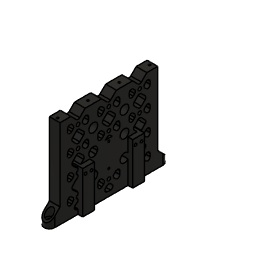
sensors-plate_front-support_rgbd-cameras (Autodesk Fusion 360 design; units mm, degrees)
Autodesk Fusion 360 part; units mm, degrees
note: some values were not read from the file. Set by a fixed rule: which face or edge a step refers to.
(part 1 of 2)
sketch "Sketch1" plane through (0, 90, 0) normal (0, 1, 0) x (-1, 0, 0)
  arc A0 (-180, -120) -> (-165, -135) centre (-165, -120) ccw
  line L0 (-165, -135) -> (165, -135)
  arc A1 (165, -135) -> (180, -120) centre (165, -120) ccw
  line L1 (180, -120) -> (180, 120)
  arc A2 (180, 120) -> (165, 135) centre (165, 120) ccw
  line L2 (165, 135) -> (-165, 135)
  arc A3 (-165, 135) -> (-180, 120) centre (-165, 120) ccw
  line L3 (-180, 120) -> (-180, -120)
  circle A4 centre (165.5, 92) radius 2
  circle A5 centre (-165.5, 92) radius 2 construction
  circle A6 centre (165.5, -92) radius 2
  circle A7 centre (-165.5, -92) radius 2 construction
  line L4 (-178, 131) -> (-180, 131)
  line L5 (-176, -131) -> (-178, -131)
  line L6 (-176, 131) -> (-178, 131)
  line L7 (-178, -131) -> (-180, -131)
  line L8 (-180, 131) -> (-180, -131)
  line L9 (-176, -133) -> (-176, -135)
  line L10 (176, -131) -> (176, -133)
  line L11 (-176, -131) -> (-176, -133)
  line L12 (176, -133) -> (176, -135)
  line L13 (-176, -135) -> (176, -135)
  line L14 (176, 133) -> (176, 135)
  line L15 (-176, 131) -> (-176, 133)
  line L16 (176, 131) -> (176, 133)
  line L17 (-176, 133) -> (-176, 135)
  line L18 (176, 135) -> (-176, 135)
  line L19 (178, -131) -> (180, -131)
  line L20 (176, 131) -> (178, 131)
  line L21 (176, -131) -> (178, -131)
  line L22 (178, 131) -> (180, 131)
  line L23 (180, -131) -> (180, 131)
  circle A8 centre (120, -60) radius 2
  circle A9 centre (0, 120) radius 2
  circle A10 centre (120, 120) radius 2
  circle A11 centre (-120, 0) radius 2
  circle A12 centre (0, -120) radius 2
  circle A13 centre (0, -60) radius 2
  circle A14 centre (165.5, 26.5835) radius 2.5
  circle A15 centre (0, 0) radius 2
  circle A16 centre (60, 120) radius 2
  circle A17 centre (-165.5, -26.5835) radius 2.5 construction
  circle A18 centre (165.5, 78.1855) radius 2.5
  circle A19 centre (120, 0) radius 2
  circle A20 centre (120, -120) radius 2
  circle A21 centre (-60, 60) radius 2
  circle A22 centre (-60, 120) radius 2
  circle A23 centre (-120, -60) radius 2
  circle A24 centre (60, 60) radius 2
  circle A25 centre (0, 60) radius 2
  circle A26 centre (165.5, -26.5835) radius 2.5
  circle A27 centre (60, -60) radius 2
  circle A28 centre (-165.5, 26.5835) radius 2.5 construction
  circle A29 centre (60, 0) radius 2
  circle A30 centre (120, 60) radius 2
  circle A31 centre (165.5, -78.1855) radius 2.5
  circle A32 centre (-120, 60) radius 2
  circle A33 centre (-120, 120) radius 2
  circle A34 centre (-60, -120) radius 2
  circle A35 centre (-165.5, 78.1855) radius 2.5 construction
  circle A36 centre (-120, -120) radius 2
  circle A37 centre (-60, 0) radius 2
  circle A38 centre (60, -120) radius 2
  circle A39 centre (-165.5, -78.1855) radius 2.5 construction
  circle A40 centre (-60, -60) radius 2
  line L24 (176, -131) -> (176, 131)
  line L25 (176, -131) -> (-176, -131)
  line L26 (-176, -131) -> (-176, 131)
  line L27 (-176, 131) -> (176, 131)
  circle A41 centre (-165.5, -92) radius 9
  circle A42 centre (-165.5, 92) radius 9
  circle A43 centre (-165.5, -92) radius 2.25
  circle A44 centre (-165.5, 92) radius 2.25
  line L28 (-156.5, -92) -> (-156.5, 92)
  line L29 (-174.5, 92) -> (-174.5, -92)
  circle A45 centre (-165.5, -78.1855) radius 1.75
  circle A46 centre (-165.5, -26.5835) radius 1.75
  circle A47 centre (-165.5, 26.5835) radius 1.75
  circle A48 centre (-165.5, 78.1855) radius 1.75
  dimension "d15" = 18
  dimension "d17" = 4.5
  dimension "d19" = 3.5
  constraint coincident L10.start L21.start
  constraint coincident L16.start L20.start
  constraint coincident L5.start L11.start
  constraint coincident L6.start L15.start
  constraint concentric A7 A41
  constraint concentric A5 A42
  constraint concentric A41 A43
  constraint concentric A42 A44
  constraint coincident A41 L28.start
  constraint coincident A42 L28.end
  constraint tangent A41 L28
  constraint tangent A42 L28
  constraint coincident A42 L29.start
  constraint coincident A41 L29.end
  constraint tangent A42 L29
  constraint tangent A41 L29
  constraint concentric A39 A45
  constraint concentric A17 A46
  constraint concentric A28 A47
  constraint concentric A35 A48
  constraint equal A45 A46
  constraint equal A45 A47
  constraint equal A45 A48
  constraint equal A41 A42
  constraint equal A43 A44
  measures "d15" diameter of A41
  measures "d17" diameter of A43
  measures "d19" diameter of A45
extrude "Extrude1" add sketch "Sketch1" along normal blind 8 contours A41 | A41 A42 L28 L29 | A42
sketch "Sketch2" plane through (0, 98, 0) normal (0, 1, 0) x (-1, 0, 0)
  circle A0 centre (-165.5, -78.1855) radius 1.75
  circle A1 centre (-165.5, -26.5835) radius 1.75
  circle A2 centre (-165.5, 92) radius 2.25
  circle A3 centre (-165.5, 78.1855) radius 1.75
  circle A4 centre (-165.5, -92) radius 2.25
  circle A5 centre (-165.5, 26.5835) radius 1.75
  line L0 (-174.5, 92) -> (-174.5, -92)
  arc A6 (-174.5, -92) -> (-156.5, -92) centre (-165.5, -92) ccw
  line L1 (-156.5, -92) -> (-156.5, 92)
  arc A7 (-156.5, 92) -> (-174.5, 92) centre (-165.5, 92) ccw
  circle A8 centre (-165.5, -92) radius 9 construction
  line L2 (-165.5, -92) -> (-165.5, -83) construction
  line L3 (-165.5, -83) -> (-156.5, -83)
  line L4 (-165.5, -83) -> (-174.5, -83)
  line L5 (-156.5, 0) -> (-174.5, 0) construction
  line L6 (-156.5, 83) -> (-174.5, 83)
  constraint concentric A4 A8
  constraint coincident A6.end A8
  constraint coincident A4.centre A6.centre
  constraint coincident A8 L2.end
  constraint vertical L2
  constraint coincident L1 L3.end
  constraint perpendicular L1 L3
  constraint coincident L0 L4.end
  constraint perpendicular L0 L4
  constraint midpoint L1 L5.start
  constraint midpoint L0 L5.end
  constraint coincident L1 L6.start
  constraint coincident L0 L6.end
  constraint perpendicular L0 L6
extrude "Extrude2" add sketch "Sketch2" along normal blind 142 contours L0 L1 L3 L4 L6
sketch "Sketch3" plane through (0, 90, 0) normal (0, -1, 0) x (1, 0, 0)
  circle A0 centre (165.5, -78.1855) radius 1.75
  circle A1 centre (165.5, -26.5835) radius 1.75
  circle A2 centre (165.5, 92) radius 2.25
  circle A3 centre (165.5, 78.1855) radius 1.75
  circle A4 centre (165.5, -92) radius 2.25
  circle A5 centre (165.5, 26.5835) radius 1.75
  line L0 (174.5, -92) -> (174.5, 92)
  arc A6 (174.5, 92) -> (156.5, 92) centre (165.5, 92) ccw
  line L1 (156.5, 92) -> (156.5, -92)
  arc A7 (156.5, -92) -> (174.5, -92) centre (165.5, -92) ccw
extrude "Extrude3" add sketch "Sketch3" against normal blind 125 contours A0 | A1 | A3 | A5
sketch "Sketch5" plane through (0, 90, 0) normal (0, -1, 0) x (1, 0, 0)
  circle A0 centre (165.5, 92) radius 2.25
  circle A1 centre (165.5, -92) radius 2.25
  line L0 (174.5, -92) -> (174.5, 92)
  arc A2 (174.5, 92) -> (156.5, 92) centre (165.5, 92) ccw
  line L1 (156.5, 92) -> (156.5, -92)
  arc A3 (156.5, -92) -> (174.5, -92) centre (165.5, -92) ccw
  circle A4 centre (165.5, -92) radius 6
  circle A5 centre (165.5, 92) radius 6
  circle A6 centre (165.5, -92) radius 9
  circle A7 centre (165.5, 92) radius 9
  line L2 (174.5, -83) -> (156.5, -83)
  line L3 (174.5, 83) -> (156.5, 83)
  dimension "d34" = 12
  constraint concentric A1 A4
  constraint concentric A0 A5
  constraint equal A4 A5
  constraint concentric A4 A6
  constraint coincident L0.start A6
  constraint concentric A5 A7
  constraint coincident L0.end A7
  constraint coincident L0 L2.start
  constraint coincident L1 L2.end
  constraint perpendicular L1 L2
  constraint tangent A6 L2
  constraint coincident L0 L3.start
  constraint coincident L1 L3.end
  constraint perpendicular L1 L3
  constraint tangent A7 L3
  measures "d34" diameter of A4
extrude "Extrude4" add sketch "Sketch5" against normal blind 26 contours L0 A6 L2 | A3 A6 | L1 A6 L2 | L0 A7 L3 | A2 A7 | L1 A7 L3
sketch "Sketch6" plane through (156.5, 0, 0) normal (-1, 0, 0) x (0, 0, 1)
  line L0 (83, 116) -> (83, 240)
  line L1 (83, 240) -> (-83, 240)
  line L2 (-83, 240) -> (-83, 116)
  line L3 (-83, 116) -> (-92, 116)
  line L4 (-92, 116) -> (-92, 90) construction
  line L5 (-92, 90) -> (92, 90)
  line L6 (92, 90) -> (92, 116) construction
  line L7 (92, 116) -> (83, 116)
  line L8 (101, 116) -> (92, 116)
  line L9 (92, 116) -> (83, 116)
  line L10 (83, 116) -> (83, 240)
  line L11 (-92, 90) -> (-101, 90)
  line L12 (92, 90) -> (-92, 90)
  line L13 (101, 90) -> (92, 90)
  line L14 (-83, 116) -> (-92, 116)
  line L15 (-92, 116) -> (-101, 116)
  line L16 (-83, 116) -> (-83, 240)
  line L17 (83, 240) -> (-83, 240)
  line L18 (101, 90) -> (101, 116)
  line L19 (-101, 90) -> (-101, 116)
  line L20 (-83, 116) -> (-101, 98)
  line L21 (-83, 116) -> (-57.5442, 116) construction
  line L22 (83, 116) -> (101, 98)
  line L23 (83, 116) -> (106.4307, 116) construction
  dimension "d37" = 135
  dimension "d38" = 45
  constraint horizontal L21
  constraint coincident L2.end L3.start
  constraint coincident L19 L20.end
  constraint horizontal L23
  constraint coincident L0.start L7.end
  constraint coincident L18 L22.end
  measures "d37" angle of L20 L21
  measures "d38" angle of L22 L23
extrude "Extrude5" cut sketch "Sketch6" against normal up to surface (18 mm away) contours L7 L8 L9 L18 L22 | L3 L14 L15 L19 L20
sketch "Sketch7" plane through (0, 240, 0) normal (0, 1, 0) x (-1, 0, 0)
  circle A0 centre (-165.5, 78.1855) radius 1.75
  circle A1 centre (-165.5, 26.5835) radius 1.75
  circle A2 centre (-165.5, -78.1855) radius 1.75
  circle A3 centre (-165.5, -26.5835) radius 1.75
  line L0 (-174.5, -83) -> (-156.5, -83)
  line L1 (-156.5, -83) -> (-156.5, 83)
  line L2 (-156.5, 83) -> (-174.5, 83)
  line L3 (-174.5, 83) -> (-174.5, -83)
  line L4 (-174.5, -70.1855) -> (-156.5, -70.1855)
  line L5 (-174.5, -34.5835) -> (-156.5, -34.5835)
  line L6 (-174.5, -18.5835) -> (-156.5, -18.5835)
  line L7 (-174.5, 18.5835) -> (-156.5, 18.5835)
  line L8 (-174.5, 34.5835) -> (-156.5, 34.5835)
  line L9 (-174.5, 70.1855) -> (-156.5, 70.1855)
  dimension "d41" = 8
  dimension "d43" = 8
  dimension "d44" = 8
  dimension "d45" = 8
  dimension "d46" = 8
  dimension "d47" = 8
  constraint coincident L3 L4.start
  constraint coincident L1 L4.end
  constraint perpendicular L1 L4
  constraint coincident L3 L5.start
  constraint coincident L1 L5.end
  constraint perpendicular L1 L5
  constraint coincident L3 L6.start
  constraint coincident L1 L6.end
  constraint perpendicular L1 L6
  constraint coincident L3 L7.start
  constraint coincident L1 L7.end
  constraint perpendicular L1 L7
  constraint coincident L3 L8.start
  constraint coincident L1 L8.end
  constraint perpendicular L1 L8
  constraint coincident L3 L9.start
  constraint coincident L1 L9.end
  constraint perpendicular L1 L9
  measures "d41" distance of A2.centre L4
  measures "d43" distance of A3.centre L5
  measures "d44" distance of A3.centre L6
  measures "d45" distance of A1.centre L7
  measures "d46" distance of A1.centre L8
  measures "d47" distance of A0.centre L9
extrude "Extrude6" cut sketch "Sketch7" against normal blind 142 contours L1 L3 L4 L5 | L1 L3 L6 L7 | L1 L3 L8 L9
sketch "Sketch8" plane through (156.5, 0, 0) normal (-1, 0, 0) x (0, 0, 1)
  line L0 (-70.1855, 98) -> (-70.1855, 240)
  line L1 (-70.1855, 240) -> (-83, 240)
  line L2 (-83, 240) -> (-83, 116)
  line L3 (-83, 116) -> (-92, 107)
  line L4 (-92, 107) -> (-92, 90)
  line L5 (-92, 90) -> (92, 90)
  line L6 (92, 90) -> (92, 107)
  line L7 (92, 107) -> (83, 116)
  line L8 (83, 116) -> (83, 240)
  line L9 (83, 240) -> (70.1855, 240)
  line L10 (70.1855, 240) -> (70.1855, 98)
  line L11 (70.1855, 98) -> (34.5835, 98)
  line L12 (34.5835, 98) -> (34.5835, 240)
  line L13 (34.5835, 240) -> (18.5835, 240)
  line L14 (18.5835, 240) -> (18.5835, 98)
  line L15 (18.5835, 98) -> (-18.5835, 98)
  line L16 (-18.5835, 98) -> (-18.5835, 240)
  line L17 (-18.5835, 240) -> (-34.5835, 240)
  line L18 (-34.5835, 240) -> (-34.5835, 98)
  line L19 (-34.5835, 98) -> (-70.1855, 98)
  line L20 (-70.1855, 169) -> (70.1855, 169) construction
  line L21 (-70.1855, 169) -> (-70.1855, 98)
  line L22 (70.1855, 169) -> (70.1855, 98)
  line L23 (70.1855, 169) -> (70.1855, 240)
  line L24 (-70.1855, 169) -> (-70.1855, 240)
  line L25 (-70.1855, 204.5) -> (70.1855, 204.5) construction
  line L26 (-70.1855, 133.5) -> (70.1855, 133.5) construction
  line L27 (-70.1855, 98) -> (-34.5835, 133.5) construction
  line L28 (-34.5835, 133.5) -> (-70.1855, 169) construction
  line L29 (-70.1855, 169) -> (-34.5835, 204.5) construction
  line L30 (-34.5835, 204.5) -> (-70.1855, 240) construction
  line L31 (-34.5835, 240) -> (-70.1855, 204.5) construction
  line L32 (-70.1855, 204.5) -> (-34.5835, 169) construction
  line L33 (-34.5835, 169) -> (-70.1855, 133.5) construction
  line L34 (-70.1855, 133.5) -> (-34.5835, 98) construction
  line L35 (-18.5835, 98) -> (18.5835, 133.5) construction
  line L36 (18.5835, 133.5) -> (-18.5835, 169) construction
  line L37 (-18.5835, 169) -> (18.5835, 204.5) construction
  line L38 (18.5835, 204.5) -> (-18.5835, 240) construction
  line L39 (18.5835, 240) -> (-18.5835, 204.5) construction
  line L40 (-18.5835, 204.5) -> (18.5835, 169) construction
  line L41 (18.5835, 169) -> (-18.5835, 133.5) construction
  line L42 (-18.5835, 133.5) -> (18.5835, 98) construction
  line L43 (34.5835, 240) -> (70.1855, 204.5) construction
  line L44 (70.1855, 204.5) -> (34.5835, 169) construction
  line L45 (34.5835, 169) -> (70.1855, 133.5) construction
  line L46 (70.1855, 133.5) -> (34.5835, 98) construction
  line L47 (70.1855, 98) -> (34.5835, 133.5) construction
  line L48 (34.5835, 133.5) -> (70.1855, 169) construction
  line L49 (70.1855, 169) -> (34.5835, 204.5) construction
  line L50 (34.5835, 204.5) -> (70.1855, 240) construction
  line L51 (15.8207, 242.8926) -> (-24.3747, 204.5)
  line L52 (-24.3747, 204.5) -> (12.7923, 169)
  line L53 (12.7923, 169) -> (-24.3747, 133.5)
  line L54 (-24.3747, 133.5) -> (15.8207, 95.1074)
  line L55 (21.3463, 237.1074) -> (-12.7923, 204.5)
  line L56 (-12.7923, 204.5) -> (24.3747, 169)
  line L57 (24.3747, 169) -> (-12.7923, 133.5)
  line L58 (-12.7923, 133.5) -> (21.3463, 100.8926)
  line L59 (-15.8207, 95.1074) -> (24.3747, 133.5)
  line L60 (24.3747, 133.5) -> (-12.7923, 169)
  line L61 (-12.7923, 169) -> (24.3747, 204.5)
  line L62 (24.3747, 204.5) -> (-15.8207, 242.8926)
  line L63 (-21.3463, 100.8926) -> (12.7923, 133.5)
  line L64 (12.7923, 133.5) -> (-24.3747, 169)
  line L65 (-24.3747, 169) -> (12.7923, 204.5)
  line L66 (12.7923, 204.5) -> (-21.3463, 237.1074)
  line L67 (-37.4079, 242.8325) -> (-75.8505, 204.5)
  line L68 (-75.8505, 204.5) -> (-40.2485, 169)
  line L69 (-40.2485, 169) -> (-75.8505, 133.5)
  line L70 (-75.8505, 133.5) -> (-37.4079, 95.1675)
  line L71 (-31.7591, 237.1675) -> (-64.5205, 204.5)
  line L72 (-64.5205, 204.5) -> (-28.9185, 169)
  line L73 (-28.9185, 169) -> (-64.5205, 133.5)
  line L74 (-64.5205, 133.5) -> (-31.7591, 100.8325)
  line L75 (-67.3611, 95.1675) -> (-28.9185, 133.5)
  line L76 (-28.9185, 133.5) -> (-64.5205, 169)
  line L77 (-64.5205, 169) -> (-28.9185, 204.5)
  line L78 (-28.9185, 204.5) -> (-67.3611, 242.8325)
  line L79 (-73.0099, 100.8325) -> (-40.2485, 133.5)
  line L80 (-40.2485, 133.5) -> (-75.8505, 169)
  line L81 (-75.8505, 169) -> (-40.2485, 204.5)
  line L82 (-40.2485, 204.5) -> (-73.0099, 237.1675)
  line L83 (73.0099, 100.8325) -> (40.2485, 133.5)
  line L84 (40.2485, 133.5) -> (75.8505, 169)
  line L85 (75.8505, 169) -> (40.2485, 204.5)
  line L86 (40.2485, 204.5) -> (73.0099, 237.1675)
  line L87 (67.3611, 95.1675) -> (28.9185, 133.5)
  line L88 (28.9185, 133.5) -> (64.5205, 169)
  line L89 (64.5205, 169) -> (28.9185, 204.5)
  line L90 (28.9185, 204.5) -> (67.3611, 242.8325)
  line L91 (31.7591, 237.1675) -> (64.5205, 204.5)
  line L92 (64.5205, 204.5) -> (28.9185, 169)
  line L93 (28.9185, 169) -> (64.5205, 133.5)
  line L94 (64.5205, 133.5) -> (31.7591, 100.8325)
  line L95 (37.4079, 242.8325) -> (75.8505, 204.5)
  line L96 (75.8505, 204.5) -> (40.2485, 169)
  line L97 (40.2485, 169) -> (75.8505, 133.5)
  line L98 (75.8505, 133.5) -> (37.4079, 95.1675)
  line L99 (-70.1855, 240) -> (70.1855, 240)
  circle A0 centre (-52.3845, 151.25) radius 3
  circle A1 centre (-52.3845, 186.75) radius 3
  circle A2 centre (-52.3845, 222.25) radius 3
  circle A3 centre (-52.3845, 115.75) radius 3
  circle A4 centre (0, 115.75) radius 3
  circle A5 centre (0, 151.25) radius 3
  circle A6 centre (0, 186.75) radius 3
  circle A7 centre (0, 222.25) radius 3
  circle A8 centre (52.3845, 222.25) radius 3
  circle A9 centre (52.3845, 186.75) radius 3
  circle A10 centre (52.3845, 151.25) radius 3
  circle A11 centre (52.3845, 115.75) radius 3
  dimension "d50" = 4
  dimension "d51" = -4
  dimension "d52" = 4
  dimension "d53" = -4
  dimension "d54" = 4
  dimension "d55" = -4
  dimension "d56" = 4
  dimension "d57" = -4
  dimension "d58" = 4
  dimension "d59" = -4
  dimension "d60" = 4
  dimension "d61" = -4
  dimension "d62" = 6
  constraint midpoint L0 L20.start
  constraint midpoint L10 L20.end
  constraint coincident L0.start L19.end
  constraint coincident L10.end L11.start
  constraint coincident L9.end L10.start
  constraint coincident L0.end L1.start
  constraint midpoint L24 L25.start
  constraint midpoint L23 L25.end
  constraint midpoint L21 L26.start
  constraint midpoint L22 L26.end
  constraint coincident L26 L27.end
  constraint coincident L18 L27.end
  constraint coincident L25 L29.end
  constraint coincident L18 L29.end
  constraint coincident L17.end L18.start
  constraint midpoint L18 L32.end
  constraint coincident L18.end L19.start
  constraint coincident L15.end L16.start
  constraint coincident L14 L35.end
  constraint coincident L26 L35.end
  constraint midpoint L16 L36.end
  constraint coincident L25 L37.end
  constraint coincident L14 L37.end
  constraint coincident L16.end L17.start
  constraint coincident L13.end L14.start
  constraint coincident L25 L39.end
  constraint coincident L16 L39.end
  constraint midpoint L14 L40.end
  constraint coincident L26 L41.end
  constraint coincident L16 L41.end
  constraint coincident L14.end L15.start
  constraint coincident L12.end L13.start
  constraint midpoint L12 L44.end
  constraint coincident L11.end L12.start
  constraint coincident L26 L47.end
  constraint coincident L12 L47.end
  constraint coincident L25 L49.end
  constraint coincident L12 L49.end
  constraint midpoint L28 A0.centre
  constraint midpoint L32 A1.centre
  constraint midpoint L31 A2.centre
  constraint midpoint L27 A3.centre
  constraint midpoint L42 A4.centre
  constraint midpoint L41 A5.centre
  constraint midpoint L40 A6.centre
  constraint midpoint L39 A7.centre
  constraint midpoint L43 A8.centre
  constraint midpoint L49 A9.centre
  constraint midpoint L48 A10.centre
  constraint midpoint L46 A11.centre
  constraint equal A0 A1
  constraint equal A0 A2
  constraint equal A0 A3
  constraint equal A3 A4
  constraint equal A3 A5
  constraint equal A0 A6
  constraint equal A1 A7
  constraint equal A7 A8
  constraint equal A6 A9
  constraint equal A5 A10
  constraint equal A4 A11
  measures "d62" diameter of A0
extrude "Extrude7" add sketch "Sketch8" against normal up to surface (18 mm away) contours L0 L19 L21 L70 L75 L79 | L0 L21 L69 L70 L73 L74 L79 L80 | L70 L74 L75 L79 | L18 L19 L70 L74 L75 | L18 L73 L74 L75 L76 L79 L80 | L0 L21 L24 L68 L69 L76 L77 L80 L81 | L69 L73 L76 L80 | L18 L68 L69 L72 L73 L76 L77 | L0 L24 L67 L68 L71 L72 L81 L82 | L68 L72 L77 L81 | L18 L71 L72 L77 L78 L81 L82 | L0 L24 L67 L78 L82 L99 | L67 L71 L78 L82 | L18 L67 L71 L78 L99 | L16 L51 L62 L66 L99 | L16 L51 L52 L55 L56 L65 L66 | L51 L55 L62 L66 | L14 L51 L55 L62 L99 | L14 L55 L56 L61 L62 L65 L66 | L16 L52 L53 L60 L61 L64 L65 | L52 L56 L61 L65 | L12 L90 L91 L95 L99 | L14 L52 L53 L56 L57 L60 L61 | L16 L53 L54 L57 L58 L63 L64 | L53 L57 L60 L64 | L12 L85 L86 L89 L90 L91 L92 | L86 L90 L91 L95 | L10 L23 L86 L90 L95 L99 | L14 L57 L58 L59 L60 L63 L64 | L10 L23 L85 L86 L91 L92 L95 L96 | L15 L16 L54 L59 L63 | L54 L58 L59 L63 | L12 L88 L89 L92 L93 L96 L97 | L85 L89 L92 L96 | L14 L15 L54 L58 L59 | L10 L22 L23 L84 L85 L88 L89 L96 L97 | L12 L83 L84 L87 L88 L93 L94 | L84 L88 L93 L97 | L10 L22 L83 L84 L93 L94 L97 L98 | L11 L12 L87 L94 L98 | L83 L87 L94 L98 | L10 L11 L22 L83 L87 L98
sketch "Sketch9" plane through (156.5, 0, 0) normal (-1, 0, 0) x (0, 0, 1)
  line L0 (70.1855, 163.3512) -> (70.1855, 139.1488)
  line L1 (70.1855, 139.1488) -> (58.0495, 151.25)
  line L2 (58.0495, 151.25) -> (70.1855, 163.3512)
  line L3 (70.1855, 174.6488) -> (58.0495, 186.75)
  line L4 (58.0495, 186.75) -> (70.1855, 198.8512)
  line L5 (70.1855, 198.8512) -> (70.1855, 174.6488)
  line L6 (70.1855, 210.1488) -> (58.0495, 222.25)
  line L7 (58.0495, 222.25) -> (70.1855, 234.3512)
  line L8 (70.1855, 234.3512) -> (70.1855, 210.1488)
  line L9 (83, 240) -> (64.5205, 240)
  line L10 (64.5205, 240) -> (52.3845, 227.8988)
  line L11 (52.3845, 227.8988) -> (40.2485, 240)
  line L12 (40.2485, 240) -> (12.7923, 240)
  line L13 (12.7923, 240) -> (0, 227.7814)
  line L14 (0, 227.7814) -> (-12.7923, 240)
  line L15 (-12.7923, 240) -> (-40.2485, 240)
  line L16 (-40.2485, 240) -> (-52.3845, 227.8988)
  line L17 (-52.3845, 227.8988) -> (-64.5205, 240)
  line L18 (-64.5205, 240) -> (-83, 240)
  line L19 (-83, 240) -> (-83, 116)
  line L20 (-83, 116) -> (-92, 107)
  line L21 (-92, 107) -> (-92, 90)
  line L22 (-92, 90) -> (92, 90)
  line L23 (92, 90) -> (92, 107)
  line L24 (92, 107) -> (83, 116)
  line L25 (83, 116) -> (83, 240)
  line L26 (34.5835, 234.3512) -> (46.7195, 222.25)
  line L27 (46.7195, 222.25) -> (34.5835, 210.1488)
  line L28 (34.5835, 210.1488) -> (34.5835, 234.3512)
  line L29 (34.5835, 198.8512) -> (46.7195, 186.75)
  line L30 (46.7195, 186.75) -> (34.5835, 174.6488)
  line L31 (34.5835, 174.6488) -> (34.5835, 198.8512)
  line L32 (34.5835, 163.3512) -> (46.7195, 151.25)
  line L33 (46.7195, 151.25) -> (34.5835, 139.1488)
  line L34 (34.5835, 139.1488) -> (34.5835, 163.3512)
  line L35 (34.5835, 127.8512) -> (46.7195, 115.75)
  line L36 (46.7195, 115.75) -> (34.5835, 103.6488)
  line L37 (34.5835, 103.6488) -> (34.5835, 127.8512)
  line L38 (40.2485, 98) -> (52.3845, 110.1012)
  line L39 (52.3845, 110.1012) -> (64.5205, 98)
  line L40 (64.5205, 98) -> (40.2485, 98)
  circle A0 centre (52.3845, 186.75) radius 3
  circle A1 centre (52.3845, 115.75) radius 3
  circle A2 centre (52.3845, 151.25) radius 3
  line L41 (52.3845, 145.6012) -> (64.5205, 133.5)
  line L42 (64.5205, 133.5) -> (52.3845, 121.3988)
  line L43 (52.3845, 121.3988) -> (40.2485, 133.5)
  line L44 (40.2485, 133.5) -> (52.3845, 145.6012)
  line L45 (52.3845, 156.8988) -> (40.2485, 169)
  line L46 (40.2485, 169) -> (52.3845, 181.1012)
  line L47 (52.3845, 181.1012) -> (64.5205, 169)
  line L48 (64.5205, 169) -> (52.3845, 156.8988)
  circle A3 centre (52.3845, 222.25) radius 3
  line L49 (52.3845, 216.6012) -> (64.5205, 204.5)
  line L50 (64.5205, 204.5) -> (52.3845, 192.3988)
  line L51 (52.3845, 192.3988) -> (40.2485, 204.5)
  line L52 (40.2485, 204.5) -> (52.3845, 216.6012)
  line L53 (18.5835, 127.9686) -> (18.5835, 103.5314)
  line L54 (18.5835, 103.5314) -> (5.7912, 115.75)
  line L55 (5.7912, 115.75) -> (18.5835, 127.9686)
  line L56 (18.5835, 139.0314) -> (5.7912, 151.25)
  line L57 (5.7912, 151.25) -> (18.5835, 163.4686)
  line L58 (18.5835, 163.4686) -> (18.5835, 139.0314)
  line L59 (18.5835, 174.5314) -> (5.7912, 186.75)
  line L60 (5.7912, 186.75) -> (18.5835, 198.9686)
  line L61 (18.5835, 198.9686) -> (18.5835, 174.5314)
  line L62 (18.5835, 210.0314) -> (5.7912, 222.25)
  line L63 (5.7912, 222.25) -> (18.5835, 234.4686)
  line L64 (18.5835, 234.4686) -> (18.5835, 210.0314)
  line L65 (70.1855, 103.6488) -> (58.0495, 115.75)
  line L66 (58.0495, 115.75) -> (70.1855, 127.8512)
  line L67 (70.1855, 127.8512) -> (70.1855, 103.6488)
  line L68 (-18.5835, 234.4686) -> (-5.7912, 222.25)
  line L69 (-5.7912, 222.25) -> (-18.5835, 210.0314)
  line L70 (-18.5835, 210.0314) -> (-18.5835, 234.4686)
  line L71 (-18.5835, 198.9686) -> (-5.7912, 186.75)
  line L72 (-5.7912, 186.75) -> (-18.5835, 174.5314)
  line L73 (-18.5835, 174.5314) -> (-18.5835, 198.9686)
  line L74 (-18.5835, 163.4686) -> (-5.7912, 151.25)
  line L75 (-5.7912, 151.25) -> (-18.5835, 139.0314)
  line L76 (-18.5835, 139.0314) -> (-18.5835, 163.4686)
  line L77 (-18.5835, 127.9686) -> (-5.7912, 115.75)
  line L78 (-5.7912, 115.75) -> (-18.5835, 103.5314)
  line L79 (-18.5835, 103.5314) -> (-18.5835, 127.9686)
  circle A4 centre (0, 222.25) radius 3
  line L80 (0, 145.7186) -> (12.7923, 133.5)
  line L81 (12.7923, 133.5) -> (0, 121.2814)
  line L82 (0, 121.2814) -> (-12.7923, 133.5)
  line L83 (-12.7923, 133.5) -> (0, 145.7186)
  line L84 (0, 156.7814) -> (-12.7923, 169)
  line L85 (-12.7923, 169) -> (0, 181.2186)
  line L86 (0, 181.2186) -> (12.7923, 169)
  line L87 (12.7923, 169) -> (0, 156.7814)
  circle A5 centre (0, 151.25) radius 3
  circle A6 centre (0, 186.75) radius 3
  circle A7 centre (0, 115.75) radius 3
  line L88 (0, 216.7186) -> (12.7923, 204.5)
  line L89 (12.7923, 204.5) -> (0, 192.2814)
  line L90 (0, 192.2814) -> (-12.7923, 204.5)
  line L91 (-12.7923, 204.5) -> (0, 216.7186)
  line L92 (-34.5835, 127.8512) -> (-34.5835, 103.6488)
  line L93 (-34.5835, 103.6488) -> (-46.7195, 115.75)
  line L94 (-46.7195, 115.75) -> (-34.5835, 127.8512)
  line L95 (-34.5835, 139.1488) -> (-46.7195, 151.25)
  line L96 (-46.7195, 151.25) -> (-34.5835, 163.3512)
  line L97 (-34.5835, 163.3512) -> (-34.5835, 139.1488)
  line L98 (-34.5835, 174.6488) -> (-46.7195, 186.75)
  line L99 (-46.7195, 186.75) -> (-34.5835, 198.8512)
  line L100 (-34.5835, 198.8512) -> (-34.5835, 174.6488)
  line L101 (-34.5835, 210.1488) -> (-46.7195, 222.25)
  line L102 (-46.7195, 222.25) -> (-34.5835, 234.3512)
  line L103 (-34.5835, 234.3512) -> (-34.5835, 210.1488)
  line L104 (-12.7923, 98) -> (0, 110.2186)
  line L105 (0, 110.2186) -> (12.7923, 98)
  line L106 (12.7923, 98) -> (-12.7923, 98)
  line L107 (-70.1855, 234.3512) -> (-58.0495, 222.25)
  line L108 (-58.0495, 222.25) -> (-70.1855, 210.1488)
  line L109 (-70.1855, 210.1488) -> (-70.1855, 234.3512)
  line L110 (-70.1855, 198.8512) -> (-58.0495, 186.75)
  line L111 (-58.0495, 186.75) -> (-70.1855, 174.6488)
  line L112 (-70.1855, 174.6488) -> (-70.1855, 198.8512)
  line L113 (-70.1855, 163.3512) -> (-58.0495, 151.25)
  line L114 (-58.0495, 151.25) -> (-70.1855, 139.1488)
  line L115 (-70.1855, 139.1488) -> (-70.1855, 163.3512)
  line L116 (-70.1855, 127.8512) -> (-58.0495, 115.75)
  line L117 (-58.0495, 115.75) -> (-70.1855, 103.6488)
  line L118 (-70.1855, 103.6488) -> (-70.1855, 127.8512)
  line L119 (-52.3845, 145.6012) -> (-40.2485, 133.5)
  line L120 (-40.2485, 133.5) -> (-52.3845, 121.3988)
  line L121 (-52.3845, 121.3988) -> (-64.5205, 133.5)
  line L122 (-64.5205, 133.5) -> (-52.3845, 145.6012)
  line L123 (-52.3845, 216.6012) -> (-40.2485, 204.5)
  line L124 (-40.2485, 204.5) -> (-52.3845, 192.3988)
  line L125 (-52.3845, 192.3988) -> (-64.5205, 204.5)
  line L126 (-64.5205, 204.5) -> (-52.3845, 216.6012)
  circle A8 centre (-52.3845, 151.25) radius 3
  line L127 (-52.3845, 156.8988) -> (-64.5205, 169)
  line L128 (-64.5205, 169) -> (-52.3845, 181.1012)
  line L129 (-52.3845, 181.1012) -> (-40.2485, 169)
  line L130 (-40.2485, 169) -> (-52.3845, 156.8988)
  circle A9 centre (-52.3845, 222.25) radius 3
  circle A10 centre (-52.3845, 186.75) radius 3
  circle A11 centre (-52.3845, 115.75) radius 3
  line L131 (-64.5205, 98) -> (-52.3845, 110.1012)
  line L132 (-52.3845, 110.1012) -> (-40.2485, 98)
  line L133 (-40.2485, 98) -> (-64.5205, 98)
  line L134 (-40.2485, 204.5) -> (-12.7923, 204.5) construction
  line L135 (-40.2485, 133.5) -> (-12.7923, 133.5) construction
  line L136 (-40.2485, 169) -> (-12.7923, 169) construction
  line L137 (12.7923, 204.5) -> (40.2485, 204.5) construction
  line L138 (12.7923, 169) -> (40.2485, 169) construction
  line L139 (12.7923, 133.5) -> (40.2485, 133.5) construction
  circle A12 centre (-26.5204, 204.5) radius 7.5
  circle A13 centre (-26.5204, 169) radius 7.5
  circle A14 centre (26.5204, 169) radius 7.5
  circle A15 centre (26.5204, 204.5) radius 7.5
  circle A16 centre (26.5204, 133.5) radius 7.5
  circle A17 centre (-26.5204, 133.5) radius 7.5
  dimension "d65" = 15
  constraint coincident L123.end L124.start
  constraint coincident L90.end L91.start
  constraint coincident L119.end L120.start
  constraint coincident L82.end L83.start
  constraint coincident L129.end L130.start
  constraint coincident L84.end L85.start
  constraint coincident L88.end L89.start
  constraint coincident L51.end L52.start
  constraint coincident L86.end L87.start
  constraint coincident L45.end L46.start
  constraint coincident L80.end L81.start
  constraint coincident L43.end L44.start
  constraint midpoint L134 A12.centre
  constraint midpoint L136 A13.centre
  constraint midpoint L138 A14.centre
  constraint midpoint L137 A15.centre
  constraint midpoint L139 A16.centre
  constraint midpoint L135 A17.centre
  constraint equal A12 A13
  constraint equal A12 A17
  constraint equal A12 A15
  constraint equal A12 A14
  constraint equal A12 A16
  measures "d65" diameter of A12
extrude "Extrude8" cut sketch "Sketch9" against normal up to surface (18 mm away) contours A12 | A13 | A14 | A15 | A16 | A17
fillet "Fillet1" radius 4 120 edges at (165.5, 192.3988, -52.3845) (165.5, 210.1488, -34.5835) (165.5, 174.6488, -34.5835) (165.5, 156.8988, -52.3845) (165.5, 139.1488, -34.5835) (165.5, 103.6488, -34.5835) (165.5, 121.3988, -52.3845) (165.5, 210.0314, 18.5835) (165.5, 192.2814, 0) (165.5, 174.5314, 18.5835) (165.5, 156.7814, 0) (165.5, 139.0314, 18.5835) (165.5, 121.2814, 0) (165.5, 103.5314, 18.5835) (165.5, 103.6488, 70.1855) (165.5, 121.3988, 52.3845) (165.5, 139.1488, 70.1855) (165.5, 156.8988, 52.3845) (165.5, 174.6488, 70.1855) (165.5, 192.3988, 52.3845) (165.5, 210.1488, 70.1855) (165.5, 210.1488, -70.1855) (165.5, 174.6488, -70.1855) (165.5, 139.1488, -70.1855) (165.5, 103.6488, -70.1855) (165.5, 103.5314, -18.5835) (165.5, 139.0314, -18.5835) (165.5, 174.5314, -18.5835) (165.5, 210.0314, -18.5835) (165.5, 210.1488, 34.5835) (165.5, 174.6488, 34.5835) (165.5, 139.1488, 34.5835) (165.5, 103.6488, 34.5835) (165.5, 234.3512, -70.1855) (165.5, 216.6012, -52.3845) (165.5, 198.8512, -70.1855) (165.5, 181.1012, -52.3845) (165.5, 163.3512, -70.1855) (165.5, 145.6012, -52.3845) (165.5, 127.8512, -70.1855) (165.5, 110.1012, -52.3845) (165.5, 234.4686, -18.5835) (165.5, 216.7186, 0) (165.5, 198.9686, -18.5835) (165.5, 181.2186, 0) (165.5, 163.4686, -18.5835) (165.5, 145.7186, 0) (165.5, 127.9686, -18.5835) (165.5, 110.2186, 0) (165.5, 234.3512, 34.5835) (165.5, 216.6012, 52.3845) (165.5, 198.8512, 34.5835) (165.5, 181.1012, 52.3845) (165.5, 163.3512, 34.5835) (165.5, 145.6012, 52.3845) (165.5, 127.8512, 34.5835) (165.5, 110.1012, 52.3845) (165.5, 234.3512, -34.5835) (165.5, 198.8512, -34.5835) (165.5, 163.3512, -34.5835) (165.5, 127.8512, -34.5835) (165.5, 127.9686, 18.5835) (165.5, 163.4686, 18.5835) (165.5, 198.9686, 18.5835) (165.5, 234.4686, 18.5835) (165.5, 234.3512, 70.1855) (165.5, 198.8512, 70.1855) (165.5, 163.3512, 70.1855) (165.5, 127.8512, 70.1855) (165.5, 204.5, -64.5205) (165.5, 169, -64.5205) (165.5, 133.5, -64.5205) (165.5, 98, -64.5205) (165.5, 204.5, -12.7923) (165.5, 169, -12.7923) (165.5, 133.5, -12.7923) (165.5, 98, -12.7923) (165.5, 204.5, 40.2485) (165.5, 169, 40.2485) (165.5, 133.5, 40.2485) (165.5, 98, 40.2485) (165.5, 222.25, -58.0495) (165.5, 186.75, -58.0495) (165.5, 151.25, -58.0495) (165.5, 115.75, -58.0495) (165.5, 133.5, -40.2485) (165.5, 169, -40.2485) (165.5, 204.5, -40.2485) (165.5, 222.25, -5.7912) (165.5, 186.75, -5.7912) (165.5, 151.25, -5.7912) (165.5, 115.75, -5.7912) (165.5, 133.5, 12.7923) (165.5, 169, 12.7923) (165.5, 204.5, 12.7923) (165.5, 98, 12.7923) (165.5, 98, -40.2485) (165.5, 98, 64.5205) (165.5, 133.5, 64.5205) (165.5, 169, 64.5205) (165.5, 204.5, 64.5205) (165.5, 222.25, 46.7195) (165.5, 186.75, 46.7195) (165.5, 151.25, 46.7195) (165.5, 115.75, 46.7195) (165.5, 222.25, 58.0495) (165.5, 186.75, 58.0495) (165.5, 151.25, 58.0495) (165.5, 115.75, 58.0495) (165.5, 222.25, 5.7912) (165.5, 186.75, 5.7912) (165.5, 151.25, 5.7912) (165.5, 115.75, 5.7912) (165.5, 115.75, -46.7195) (165.5, 151.25, -46.7195) (165.5, 186.75, -46.7195) (165.5, 222.25, -46.7195) (165.5, 227.8988, -52.3845) (165.5, 227.7814, 0) (165.5, 227.8988, 52.3845)
sketch "Sketch11" plane through (174.5, 0, 0) normal (1, 0, 0) x (0, 0, -1)
  circle A0 centre (-26.5204, 133.5) radius 7.5 construction
  circle A1 centre (26.5204, 204.5) radius 7.5 construction
  circle A2 centre (-26.5204, 169) radius 7.5 construction
  circle A3 centre (26.5204, 133.5) radius 7.5 construction
  circle A4 centre (26.5204, 169) radius 7.5 construction
  circle A5 centre (-26.5204, 204.5) radius 7.5 construction
  line L0 (-70.1855, 184.2861) -> (-70.1855, 189.2139) construction
  arc A6 (-63.3611, 192.0464) -> (-70.1855, 189.2139) centre (-66.1855, 189.2139) ccw construction
  line L1 (-63.3611, 192.0464) -> (-60.8901, 189.5825) construction
  arc A7 (-60.8901, 183.9175) -> (-60.8901, 189.5825) centre (-63.7145, 186.75) ccw construction
  line L2 (-60.8901, 183.9175) -> (-63.3611, 181.4536) construction
  arc A8 (-70.1855, 184.2861) -> (-63.3611, 181.4536) centre (-66.1855, 184.2861) ccw construction
  line L3 (-70.1855, 219.7861) -> (-70.1855, 224.7139) construction
  arc A9 (-63.3611, 227.5464) -> (-70.1855, 224.7139) centre (-66.1855, 224.7139) ccw construction
  line L4 (-63.3611, 227.5464) -> (-60.8901, 225.0825) construction
  arc A10 (-60.8901, 219.4175) -> (-60.8901, 225.0825) centre (-63.7145, 222.25) ccw construction
  line L5 (-60.8901, 219.4175) -> (-63.3611, 216.9536) construction
  arc A11 (-70.1855, 219.7861) -> (-63.3611, 216.9536) centre (-66.1855, 219.7861) ccw construction
  line L6 (-64.5205, 240) -> (-83, 240) construction
  line L7 (-83, 240) -> (-83, 116) construction
  line L8 (-83, 116) -> (-92, 107) construction
  line L9 (-92, 107) -> (-92, 90) construction
  line L10 (-92, 90) -> (92, 90) construction
  line L11 (92, 90) -> (92, 107) construction
  line L12 (92, 107) -> (83, 116) construction
  line L13 (83, 116) -> (83, 240) construction
  line L14 (83, 240) -> (64.5205, 240) construction
  line L15 (64.5205, 240) -> (55.2089, 230.715) construction
  arc A12 (49.5601, 230.715) -> (55.2089, 230.715) centre (52.3845, 233.5475) ccw construction
  line L16 (49.5601, 230.715) -> (40.2485, 240) construction
  line L17 (40.2485, 240) -> (12.7923, 240) construction
  line L18 (12.7923, 240) -> (2.7628, 230.4203) construction
  arc A13 (-2.7628, 230.4203) -> (2.7628, 230.4203) centre (0, 233.3129) ccw construction
  line L19 (-2.7628, 230.4203) -> (-12.7923, 240) construction
  line L20 (-12.7923, 240) -> (-40.2485, 240) construction
  line L21 (-40.2485, 240) -> (-49.5601, 230.715) construction
  arc A14 (-55.2089, 230.715) -> (-49.5601, 230.715) centre (-52.3845, 233.5475) ccw construction
  line L22 (-55.2089, 230.715) -> (-64.5205, 240) construction
  line L23 (-34.5835, 224.7139) -> (-34.5835, 219.7861) construction
  arc A15 (-41.4079, 216.9536) -> (-34.5835, 219.7861) centre (-38.5835, 219.7861) ccw construction
  line L24 (-41.4079, 216.9536) -> (-43.8789, 219.4175) construction
  arc A16 (-43.8789, 225.0825) -> (-43.8789, 219.4175) centre (-41.0545, 222.25) ccw construction
  line L25 (-43.8789, 225.0825) -> (-41.4079, 227.5464) construction
  arc A17 (-34.5835, 224.7139) -> (-41.4079, 227.5464) centre (-38.5835, 224.7139) ccw construction
  line L26 (-34.5835, 189.2139) -> (-34.5835, 184.2861) construction
  arc A18 (-41.4079, 181.4536) -> (-34.5835, 184.2861) centre (-38.5835, 184.2861) ccw construction
  line L27 (-41.4079, 181.4536) -> (-43.8789, 183.9175) construction
  arc A19 (-43.8789, 189.5825) -> (-43.8789, 183.9175) centre (-41.0545, 186.75) ccw construction
  line L28 (-43.8789, 189.5825) -> (-41.4079, 192.0464) construction
  arc A20 (-34.5835, 189.2139) -> (-41.4079, 192.0464) centre (-38.5835, 189.2139) ccw construction
  line L29 (-34.5835, 153.7139) -> (-34.5835, 148.7861) construction
  arc A21 (-41.4079, 145.9536) -> (-34.5835, 148.7861) centre (-38.5835, 148.7861) ccw construction
  line L30 (-41.4079, 145.9536) -> (-43.8789, 148.4175) construction
  arc A22 (-43.8789, 154.0825) -> (-43.8789, 148.4175) centre (-41.0545, 151.25) ccw construction
  line L31 (-43.8789, 154.0825) -> (-41.4079, 156.5464) construction
  arc A23 (-34.5835, 153.7139) -> (-41.4079, 156.5464) centre (-38.5835, 153.7139) ccw construction
  line L32 (-34.5835, 118.2139) -> (-34.5835, 113.2861) construction
  arc A24 (-41.4079, 110.4536) -> (-34.5835, 113.2861) centre (-38.5835, 113.2861) ccw construction
  line L33 (-41.4079, 110.4536) -> (-43.8789, 112.9175) construction
  arc A25 (-43.8789, 118.5825) -> (-43.8789, 112.9175) centre (-41.0545, 115.75) ccw construction
  line L34 (-43.8789, 118.5825) -> (-41.4079, 121.0464) construction
  arc A26 (-34.5835, 118.2139) -> (-41.4079, 121.0464) centre (-38.5835, 118.2139) ccw construction
  line L35 (-49.925, 98) -> (-54.844, 98) construction
  arc A27 (-57.6684, 104.8325) -> (-54.844, 98) centre (-54.844, 102) ccw construction
  line L36 (-57.6684, 104.8325) -> (-55.2089, 107.285) construction
  arc A28 (-49.5601, 107.285) -> (-55.2089, 107.285) centre (-52.3845, 104.4525) ccw construction
  line L37 (-49.5601, 107.285) -> (-47.1006, 104.8325) construction
  arc A29 (-49.925, 98) -> (-47.1006, 104.8325) centre (-49.925, 102) ccw construction
  line L38 (-70.1855, 113.2861) -> (-70.1855, 118.2139) construction
  arc A30 (-63.3611, 121.0464) -> (-70.1855, 118.2139) centre (-66.1855, 118.2139) ccw construction
  line L39 (-63.3611, 121.0464) -> (-60.8901, 118.5825) construction
  arc A31 (-60.8901, 112.9175) -> (-60.8901, 118.5825) centre (-63.7145, 115.75) ccw construction
  line L40 (-60.8901, 112.9175) -> (-63.3611, 110.4536) construction
  arc A32 (-70.1855, 113.2861) -> (-63.3611, 110.4536) centre (-66.1855, 113.2861) ccw construction
  circle A33 centre (-52.3845, 222.25) radius 3 construction
  line L41 (-43.0891, 166.1675) -> (-49.5601, 159.715) construction
  arc A34 (-55.2089, 159.715) -> (-49.5601, 159.715) centre (-52.3845, 162.5475) ccw construction
  line L42 (-55.2089, 159.715) -> (-61.6799, 166.1675) construction
  arc A35 (-61.6799, 171.8325) -> (-61.6799, 166.1675) centre (-58.8555, 169) ccw construction
  line L43 (-61.6799, 171.8325) -> (-55.2089, 178.285) construction
  arc A36 (-49.5601, 178.285) -> (-55.2089, 178.285) centre (-52.3845, 175.4525) ccw construction
  line L44 (-49.5601, 178.285) -> (-43.0891, 171.8325) construction
  arc A37 (-43.0891, 166.1675) -> (-43.0891, 171.8325) centre (-45.9135, 169) ccw construction
  circle A38 centre (-52.3845, 115.75) radius 3 construction
  circle A39 centre (-52.3845, 151.25) radius 3 construction
  line L45 (-61.6799, 207.3325) -> (-55.2089, 213.785) construction
  arc A40 (-49.5601, 213.785) -> (-55.2089, 213.785) centre (-52.3845, 210.9525) ccw construction
  line L46 (-49.5601, 213.785) -> (-43.0891, 207.3325) construction
  arc A41 (-43.0891, 201.6675) -> (-43.0891, 207.3325) centre (-45.9135, 204.5) ccw construction
  line L47 (-43.0891, 201.6675) -> (-49.5601, 195.215) construction
  arc A42 (-55.2089, 195.215) -> (-49.5601, 195.215) centre (-52.3845, 198.0475) ccw construction
  line L48 (-55.2089, 195.215) -> (-61.6799, 201.6675) construction
  arc A43 (-61.6799, 207.3325) -> (-61.6799, 201.6675) centre (-58.8555, 204.5) ccw construction
  line L49 (-61.6799, 136.3325) -> (-55.2089, 142.785) construction
  arc A44 (-49.5601, 142.785) -> (-55.2089, 142.785) centre (-52.3845, 139.9525) ccw construction
  line L50 (-49.5601, 142.785) -> (-43.0891, 136.3325) construction
  arc A45 (-43.0891, 130.6675) -> (-43.0891, 136.3325) centre (-45.9135, 133.5) ccw construction
  line L51 (-43.0891, 130.6675) -> (-49.5601, 124.215) construction
  arc A46 (-55.2089, 124.215) -> (-49.5601, 124.215) centre (-52.3845, 127.0475) ccw construction
  line L52 (-55.2089, 124.215) -> (-61.6799, 130.6675) construction
  arc A47 (-61.6799, 136.3325) -> (-61.6799, 130.6675) centre (-58.8555, 133.5) ccw construction
  circle A48 centre (-52.3845, 186.75) radius 3 construction
  line L53 (-18.5835, 148.3835) -> (-18.5835, 154.1165) construction
  arc A49 (-11.8207, 157.0091) -> (-18.5835, 154.1165) centre (-14.5835, 154.1165) ccw construction
  line L54 (-11.8207, 157.0091) -> (-8.8196, 154.1426) construction
  arc A50 (-8.8196, 148.3574) -> (-8.8196, 154.1426) centre (-11.5824, 151.25) ccw construction
  line L55 (-8.8196, 148.3574) -> (-11.8207, 145.4909) construction
  arc A51 (-18.5835, 148.3835) -> (-11.8207, 145.4909) centre (-14.5835, 148.3835) ccw construction
  line L56 (-18.5835, 183.8835) -> (-18.5835, 189.6165) construction
  arc A52 (-11.8207, 192.5091) -> (-18.5835, 189.6165) centre (-14.5835, 189.6165) ccw construction
  line L57 (-11.8207, 192.5091) -> (-8.8196, 189.6426) construction
  arc A53 (-8.8196, 183.8574) -> (-8.8196, 189.6426) centre (-11.5824, 186.75) ccw construction
  line L58 (-8.8196, 183.8574) -> (-11.8207, 180.9909) construction
  arc A54 (-18.5835, 183.8835) -> (-11.8207, 180.9909) centre (-14.5835, 183.8835) ccw construction
  line L59 (-18.5835, 219.3835) -> (-18.5835, 225.1165) construction
  arc A55 (-11.8207, 228.0091) -> (-18.5835, 225.1165) centre (-14.5835, 225.1165) ccw construction
  line L60 (-11.8207, 228.0091) -> (-8.8196, 225.1426) construction
  arc A56 (-8.8196, 219.3574) -> (-8.8196, 225.1426) centre (-11.5824, 222.25) ccw construction
  line L61 (-8.8196, 219.3574) -> (-11.8207, 216.4909) construction
  arc A57 (-18.5835, 219.3835) -> (-11.8207, 216.4909) centre (-14.5835, 219.3835) ccw construction
  line L62 (-60.8901, 148.4175) -> (-63.3611, 145.9536) construction
  arc A58 (-70.1855, 148.7861) -> (-63.3611, 145.9536) centre (-66.1855, 148.7861) ccw construction
  line L63 (-70.1855, 148.7861) -> (-70.1855, 153.7139) construction
  arc A59 (-63.3611, 156.5464) -> (-70.1855, 153.7139) centre (-66.1855, 153.7139) ccw construction
  line L64 (-63.3611, 156.5464) -> (-60.8901, 154.0825) construction
  arc A60 (-60.8901, 148.4175) -> (-60.8901, 154.0825) centre (-63.7145, 151.25) ccw construction
  line L65 (18.5835, 225.1165) -> (18.5835, 219.3835) construction
  arc A61 (11.8207, 216.4909) -> (18.5835, 219.3835) centre (14.5835, 219.3835) ccw construction
  line L66 (11.8207, 216.4909) -> (8.8196, 219.3574) construction
  arc A62 (8.8196, 225.1426) -> (8.8196, 219.3574) centre (11.5824, 222.25) ccw construction
  line L67 (8.8196, 225.1426) -> (11.8207, 228.0091) construction
  arc A63 (18.5835, 225.1165) -> (11.8207, 228.0091) centre (14.5835, 225.1165) ccw construction
  line L68 (18.5835, 189.6165) -> (18.5835, 183.8835) construction
  arc A64 (11.8207, 180.9909) -> (18.5835, 183.8835) centre (14.5835, 183.8835) ccw construction
  line L69 (11.8207, 180.9909) -> (8.8196, 183.8574) construction
  arc A65 (8.8196, 189.6426) -> (8.8196, 183.8574) centre (11.5824, 186.75) ccw construction
  line L70 (8.8196, 189.6426) -> (11.8207, 192.5091) construction
  arc A66 (18.5835, 189.6165) -> (11.8207, 192.5091) centre (14.5835, 189.6165) ccw construction
  line L71 (18.5835, 154.1165) -> (18.5835, 148.3835) construction
  arc A67 (11.8207, 145.4909) -> (18.5835, 148.3835) centre (14.5835, 148.3835) ccw construction
  line L72 (11.8207, 145.4909) -> (8.8196, 148.3574) construction
  arc A68 (8.8196, 154.1426) -> (8.8196, 148.3574) centre (11.5824, 151.25) ccw construction
  line L73 (8.8196, 154.1426) -> (11.8207, 157.0091) construction
  arc A69 (18.5835, 154.1165) -> (11.8207, 157.0091) centre (14.5835, 154.1165) ccw construction
  line L74 (18.5835, 118.6165) -> (18.5835, 112.8835) construction
  arc A70 (11.8207, 109.9909) -> (18.5835, 112.8835) centre (14.5835, 112.8835) ccw construction
  line L75 (11.8207, 109.9909) -> (8.8196, 112.8574) construction
  arc A71 (8.8196, 118.6426) -> (8.8196, 112.8574) centre (11.5824, 115.75) ccw construction
  line L76 (8.8196, 118.6426) -> (11.8207, 121.5091) construction
  arc A72 (18.5835, 118.6165) -> (11.8207, 121.5091) centre (14.5835, 118.6165) ccw construction
  line L77 (2.8133, 98) -> (-2.8133, 98) construction
  arc A73 (-5.5761, 104.8926) -> (-2.8133, 98) centre (-2.8133, 102) ccw construction
  line L78 (-5.5761, 104.8926) -> (-2.7628, 107.5797) construction
  arc A74 (2.7628, 107.5797) -> (-2.7628, 107.5797) centre (0, 104.6871) ccw construction
  line L79 (2.7628, 107.5797) -> (5.5761, 104.8926) construction
  arc A75 (2.8133, 98) -> (5.5761, 104.8926) centre (2.8133, 102) ccw construction
  line L80 (-9.7639, 207.3926) -> (-2.7628, 214.0797) construction
  arc A76 (2.7628, 214.0797) -> (-2.7628, 214.0797) centre (0, 211.1871) ccw construction
  line L81 (2.7628, 214.0797) -> (9.7639, 207.3926) construction
  arc A77 (9.7639, 201.6074) -> (9.7639, 207.3926) centre (7.0011, 204.5) ccw construction
  line L82 (9.7639, 201.6074) -> (2.7628, 194.9203) construction
  arc A78 (-2.7628, 194.9203) -> (2.7628, 194.9203) centre (0, 197.8129) ccw construction
  line L83 (-2.7628, 194.9203) -> (-9.7639, 201.6074) construction
  arc A79 (-9.7639, 207.3926) -> (-9.7639, 201.6074) centre (-7.0011, 204.5) ccw construction
  circle A80 centre (0, 151.25) radius 3 construction
  circle A81 centre (0, 222.25) radius 3 construction
  line L84 (9.7639, 166.1074) -> (2.7628, 159.4203) construction
  arc A82 (-2.7628, 159.4203) -> (2.7628, 159.4203) centre (0, 162.3129) ccw construction
  line L85 (-2.7628, 159.4203) -> (-9.7639, 166.1074) construction
  arc A83 (-9.7639, 171.8926) -> (-9.7639, 166.1074) centre (-7.0011, 169) ccw construction
  line L86 (-9.7639, 171.8926) -> (-2.7628, 178.5797) construction
  arc A84 (2.7628, 178.5797) -> (-2.7628, 178.5797) centre (0, 175.6871) ccw construction
  line L87 (2.7628, 178.5797) -> (9.7639, 171.8926) construction
  arc A85 (9.7639, 166.1074) -> (9.7639, 171.8926) centre (7.0011, 169) ccw construction
  circle A86 centre (0, 186.75) radius 3 construction
  line L88 (-9.7639, 136.3926) -> (-2.7628, 143.0797) construction
  arc A87 (2.7628, 143.0797) -> (-2.7628, 143.0797) centre (0, 140.1871) ccw construction
  line L89 (2.7628, 143.0797) -> (9.7639, 136.3926) construction
  arc A88 (9.7639, 130.6074) -> (9.7639, 136.3926) centre (7.0011, 133.5) ccw construction
  line L90 (9.7639, 130.6074) -> (2.7628, 123.9203)
  arc A89 (-2.7628, 123.9203) -> (2.7628, 123.9203) centre (0, 126.8129) ccw
  line L91 (-2.7628, 123.9203) -> (-9.7639, 130.6074)
  arc A90 (-9.7639, 136.3926) -> (-9.7639, 130.6074) centre (-7.0011, 133.5) ccw construction
  circle A91 centre (0, 115.75) radius 3 construction
  line L92 (34.5835, 148.7861) -> (34.5835, 153.7139) construction
  arc A92 (41.4079, 156.5464) -> (34.5835, 153.7139) centre (38.5835, 153.7139) ccw construction
  line L93 (41.4079, 156.5464) -> (43.8789, 154.0825) construction
  arc A93 (43.8789, 148.4175) -> (43.8789, 154.0825) centre (41.0545, 151.25) ccw construction
  line L94 (43.8789, 148.4175) -> (41.4079, 145.9536) construction
  arc A94 (34.5835, 148.7861) -> (41.4079, 145.9536) centre (38.5835, 148.7861) ccw construction
  line L95 (34.5835, 184.2861) -> (34.5835, 189.2139) construction
  arc A95 (41.4079, 192.0464) -> (34.5835, 189.2139) centre (38.5835, 189.2139) ccw construction
  line L96 (41.4079, 192.0464) -> (43.8789, 189.5825) construction
  arc A96 (43.8789, 183.9175) -> (43.8789, 189.5825) centre (41.0545, 186.75) ccw construction
  line L97 (43.8789, 183.9175) -> (41.4079, 181.4536) construction
  arc A97 (34.5835, 184.2861) -> (41.4079, 181.4536) centre (38.5835, 184.2861) ccw construction
  line L98 (34.5835, 219.7861) -> (34.5835, 224.7139) construction
  arc A98 (41.4079, 227.5464) -> (34.5835, 224.7139) centre (38.5835, 224.7139) ccw construction
  line L99 (41.4079, 227.5464) -> (43.8789, 225.0825) construction
  arc A99 (43.8789, 219.4175) -> (43.8789, 225.0825) centre (41.0545, 222.25) ccw construction
  line L100 (43.8789, 219.4175) -> (41.4079, 216.9536) construction
  arc A100 (34.5835, 219.7861) -> (41.4079, 216.9536) centre (38.5835, 219.7861) ccw construction
  line L101 (-8.8196, 112.8574) -> (-11.8207, 109.9909) construction
  arc A101 (-18.5835, 112.8835) -> (-11.8207, 109.9909) centre (-14.5835, 112.8835) ccw construction
  line L102 (-18.5835, 112.8835) -> (-18.5835, 118.6165) construction
  arc A102 (-11.8207, 121.5091) -> (-18.5835, 118.6165) centre (-14.5835, 118.6165) ccw construction
  line L103 (-11.8207, 121.5091) -> (-8.8196, 118.6426) construction
  arc A103 (-8.8196, 112.8574) -> (-8.8196, 118.6426) centre (-11.5824, 115.75) ccw construction
  line L104 (70.1855, 224.7139) -> (70.1855, 219.7861) construction
  arc A104 (63.3611, 216.9536) -> (70.1855, 219.7861) centre (66.1855, 219.7861) ccw construction
  line L105 (63.3611, 216.9536) -> (60.8901, 219.4175) construction
  arc A105 (60.8901, 225.0825) -> (60.8901, 219.4175) centre (63.7145, 222.25) ccw construction
  line L106 (60.8901, 225.0825) -> (63.3611, 227.5464) construction
  arc A106 (70.1855, 224.7139) -> (63.3611, 227.5464) centre (66.1855, 224.7139) ccw construction
  line L107 (70.1855, 189.2139) -> (70.1855, 184.2861) construction
  arc A107 (63.3611, 181.4536) -> (70.1855, 184.2861) centre (66.1855, 184.2861) ccw construction
  line L108 (63.3611, 181.4536) -> (60.8901, 183.9175) construction